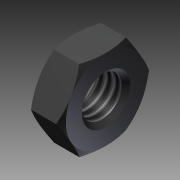
# Autodesk Inventor part: U-12-16
Saved by Autodesk Inventor 2011 SP1 (Build 150282100, 282)
## iProperties
Created: 2018-01-08
Part Number: U-12-16
Catalog Web Link: www.cadenas.de
Description: Mod. U-Iston Rod Lock Nut
Vendor: CAMOZZI
Document SubType Name: Modeling
Designer: psAdmin
Manufacturer: CAMOZZI
Mass: 0.263423 g
Surface Area: 3.18427 cm^2
Volume: 0.263423 cm^3
Density: 1 g/cm^3
Category: PARTsolutions
Company: CAMOZZI
Title: U-12-16
Author: Cadenas PARTsolutions
Comments: Iston Rod Lock Nut
PSOL_IDENT_0: {$CADENAS_DATA\23d-libs\camozzi\movimento\cilindri_a_norma_e_cilindri_standard\minicilindri_serie_16
PSOL_IDENT_1: _24_25\accessori\dado_stelo_mod_u.prj},156 {VTYP=3D},{NB=U-12-16},{LINA=U-12-16},{NN=Mod. U},{DATE=2
PSOL_IDENT_2: 7.07.2017 08:45:30},{GEOMDATE=01.02.2017 09:46:00},{VERSION=},{LINEID=20},{LINESUBID=-1},{WBVAR=}  {
PSOL_IDENT_3: NB=U-12-16},{LINA=U-12-16},{KT=DUMMY},{IDNR=},{MOD=U-12-16},{PHY=12 - 16},{D=M6x1},{M=4},{SW=10},{DN
PSOL_IDENT_4: DM=6.0},{DKDM=4.91746},{P=1.00},{INFO=Infotext}
NN: Mod. U
NT: Iston Rod Lock Nut
NB: U-12-16
NBSYN: $MOD.
LINA: U-12-16
MOD: U-12-16
PHY: 12 - 16
D: M6x1
M: 4
SW: 10
INFO: Infotext
SUPPLIER: CAMOZZI
ARTICLENO: U-12-16
BOMINFO: U-12-16
CREATOR: CADENAS GmbH
Autodesk Inventor part; units mm, degrees
sketch "Skizze_1" plane through (0, 0, 0) normal (0, 0, 1) x (1, 0, 0)
  line L0 (4, 0) -> (0, 0)
  line L1 (0, 0) -> (0, 5)
  line L2 (0, 5) -> (0.5774, 6)
  line L3 (0.5774, 6) -> (3.4226, 6)
  line L4 (3.4226, 6) -> (4, 5)
  line L5 (4, 5) -> (4, 0)
  line L6 (4, 0) -> (0, 0)
  constraints: 14 end point
revolve "Revolution1" add sketch "Skizze_1" angle 360 about axis through (4, 0, 0) along (1, 0, 0)
sketch "Skizze_2_ALT_Drilling_1" plane through (0, 0, 0) normal (0, 0, 1) x (1, 0, 0)
  line L0 (4, 0) -> (0, 0)
  line L1 (0, 0) -> (0, 3)
  line L2 (0, 3) -> (0.5415, 2.4585)
  line L3 (0.5415, 2.4585) -> (3.4585, 2.4585)
  line L4 (3.4585, 2.4585) -> (4, 3)
  line L5 (4, 3) -> (4, 0)
  line L6 (4, 0) -> (0, 0)
  constraints: 14 end point
revolve "Revolution2" cut sketch "Skizze_2_ALT_Drilling_1" angle 360 about axis through (4, 0, 0) along (1, 0, 0)
thread "Thread1" size "M6x1" class "6H" standard "ISO Metric profile" full length
sketch "Skizze_3" plane through (0, 0, 0) normal (1, 0, 0) x (0, 1, 0)
  line L0 (-10, 10) -> (-10, -10)
  line L1 (-10, -10) -> (10, -10)
  line L2 (10, -10) -> (10, 10)
  line L3 (10, 10) -> (-10, 10)
  line L4 (-2.8868, 5) -> (-5.7735, 0)
  line L5 (-5.7735, 0) -> (-2.8868, -5)
  line L6 (-2.8868, -5) -> (2.8868, -5)
  line L7 (2.8868, -5) -> (5.7735, 0)
  line L8 (5.7735, 0) -> (2.8868, 5)
  line L9 (2.8868, 5) -> (-2.8868, 5)
  constraints: 20 end point
extrude "Extrusion1" cut sketch "Skizze_3" along normal blind 4
ref_plane "DADO1_XY" through (0, 0, 0) normal (1, 0, 0) x (0, 0, -1)
ref_plane "DADO1_YZ" through (0, 0, 0) normal (0, 0, -1) x (0, 1, 0)
ref_plane "DADO1_ZX" through (0, 0, 0) normal (0, 1, 0) x (1, 0, 0)
body "Solid1"
